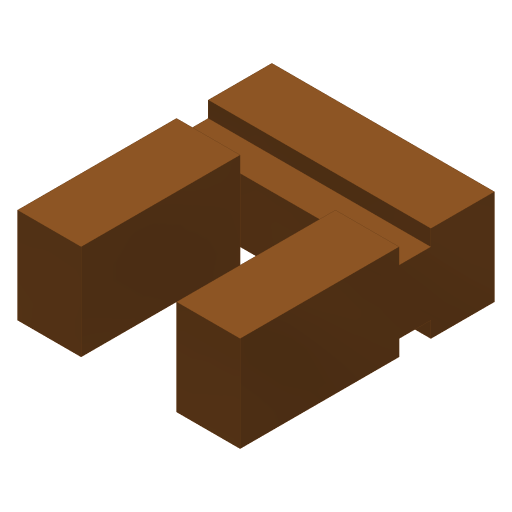
# Autodesk Inventor part: Leistende Kontakt
Saved by Autodesk Inventor 2023 (Build 270158000, 158)
## iProperties
Created: 2025-01-24
Part Number: Leistende Kontakt
Material: 2.0401 CuZn39 Pb 3 (Messing)
Document SubType Name: Modeling
Designer: abdel
Density: 8.2 g/cm^3
Appearance: Metall - Bronze(poliert)
Author: abdel
Autodesk Inventor part; units mm, degrees
ref_plane "YZ Plane" through (0, 0, 0) normal (1, 0, 0) x (0, 1, 0)
ref_plane "XZ Plane" through (0, 0, 0) normal (0, 1, 0) x (-1, 0, 0)
ref_plane "XY Plane" through (0, 0, 0) normal (0, 0, 1) x (1, 0, 0)
sketch "Skizze1" plane through (0, 0, 0) normal (0, 0, 1) x (1, 0, 0)
  line L0 (-3.5, 3) -> (3.5, 3)
  line L1 (3.5, 3) -> (3.5, 0)
  line L2 (1.5, 0) -> (-1.5, 0)
  line L3 (-3.5, 0) -> (-3.5, 3)
  line L4 (-1.5, 0) -> (-1.5, -5)
  line L5 (-1.5, -5) -> (-3.5, -5)
  line L6 (-3.5, -5) -> (-3.5, 0)
  line L7 (1.5, -5) -> (3.5, -5)
  line L8 (3.5, -5) -> (3.5, 0)
  line L9 (1.5, 0) -> (1.5, -5)
  point P0 (0, 0)
  point P1 (0, 0)
  dimension "d1" = 5
  dimension "d2" = 7
  dimension "d3" = 2
  dimension "d7" = 0
  dimension "d8" = 5
  dimension "d9" = 2
  dimension "d24" = 3
  constraints: 20 end point, 4 parallel, 2 horizontal, 2 perpendicular, 2 vertical, 1 coincident, 1 midpoint
  measures "d1" distance between parallel lines of L2 L5
  measures "d2" distance of L0.start L0.end
  measures "d3" distance of L4.end L5.end
  measures "d7" distance from line of L3.start L2
  measures "d8" distance of L2.start L7.start
  measures "d9" distance of L7.start L7.end
  measures "d24" distance between parallel lines of L2 L0
extrude "Extrusion1" add sketch "Skizze1" along normal blind 3
sketch "Skizze2" plane through (0, 0, 3) normal (0, 0, 1) x (1, 0, 0)
  line L0 (3.5, -5) -> (3.5, 3) projected
  line L1 (-3.5, 3) -> (-3.5, -5) projected
  line L2 (-3.5, 0) -> (-1.5, 0)
  line L3 (1.5, 0) -> (3.5, 0)
  line L4 (-3.5, 1) -> (3.5, 1)
  line L5 (3.5, 0) -> (3.5, 1)
  line L6 (-3.5, 0) -> (-3.5, 1)
  line L7 (-1.5, 0) -> (1.5, 0)
  point P0 (0, 0)
  dimension "d20" = 1
  constraints: 12 end point, 5 point on line, 3 horizontal, 2 vertical
  measures "d20" distance between parallel lines of L4 L3
extrude "Extrusion3" cut sketch "Skizze2" against normal blind 0.5
sketch "Skizze5" plane through (0, 0, 0) normal (0, 0, -1) x (-1, 0, 0)
  line L0 (1.5, 0) -> (-1.5, 0) projected
  line L1 (3.5, 3) -> (3.5, -5) projected
  line L2 (-3.5, -5) -> (-3.5, 3) projected
  line L3 (-3.5, 1) -> (3.5, 1)
  line L4 (3.5, 1) -> (3.5, 0)
  line L5 (3.5, 0) -> (-3.5, 0)
  line L6 (-3.5, 0) -> (-3.5, 1)
  point P0 (0, 0)
  point P1 (0, 0)
  dimension "d25" = 1
  constraints: 8 end point, 2 midpoint, 2 parallel, 2 point on line, 1 horizontal, 1 perpendicular
  measures "d25" distance between parallel lines of L3 L5
extrude "Extrusion5" cut sketch "Skizze5" against normal blind 0.5
